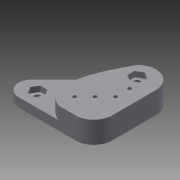
# Autodesk Inventor part: joint1+ax12imprint
Saved by Autodesk Inventor 2014 (Build 180170000, 170)
## iProperties
Created: 2014-01-13
Part Number: joint1+ax12imprint
Material: Générique
Document SubType Name: Modeling
Designer: helly
Density: 1 g/cm^3
Appearance: Par défaut
Author: helly
Autodesk Inventor part; units mm, degrees
ref_plane "YZ Plane" through (0, 0, 0) normal (1, 0, 0) x (0, 1, 0)
ref_plane "XZ Plane" through (0, 0, 0) normal (0, 1, 0) x (-1, 0, 0)
ref_plane "XY Plane" through (0, 0, 0) normal (0, 0, 1) x (1, 0, 0)
sketch "Esquisse1" plane through (0, 0, 0) normal (0, 0, 1) x (1, 0, 0)
  line L0 (0, 0) -> (52, 0) construction
  line L1 (0, 0) -> (25.4558, 25.4558) construction
  line L2 (0, 0) -> (-9.5459, 9.5459) construction
  line L3 (-9.5459, 9.5459) -> (-4.9497, 14.1421) construction
  line L4 (-4.9497, 14.1421) -> (0.7071, 19.799) construction
  line L5 (0.7071, 19.799) -> (6.364, 25.4558) construction
  line L6 (6.364, 25.4558) -> (12.0208, 31.1127) construction
  line L7 (25.4558, 25.4558) -> (19.799, 31.1127) construction
  line L8 (0, 0) -> (27.5772, 27.5772) construction
  circle A0 centre (0.7071, 19.799) radius 1 construction
  circle A1 centre (6.364, 25.4558) radius 1 construction
  circle A2 centre (12.0208, 31.1127) radius 1 construction
  circle A3 centre (19.799, 31.1127) radius 1 construction
  circle A4 centre (19.799, 0.7071) radius 1
  circle A5 centre (25.4558, 6.364) radius 1
  circle A6 centre (31.1127, 12.0208) radius 1
  circle A7 centre (31.1127, 19.799) radius 1
  circle A8 centre (27.5772, 27.5772) radius 2
  circle A9 centre (0, 0) radius 2
  line L9 (0, 0) -> (0, -8) construction
  line L10 (31.1127, 12.0208) -> (39.1127, 12.0208) construction
  line L11 (39.1127, 50.4264) -> (39.1127, -8)
  line L12 (0, 0) -> (-5.6569, 5.6569) construction
  line L13 (39.1127, -8) -> (-19.3137, -8)
  line L14 (-19.3137, -8) -> (39.1127, 50.4264)
  dimension "d31" = 45
  dimension "d32" = 13.5
  dimension "d33" = 6.5
  dimension "d34" = 8
  dimension "d35" = 8
  dimension "d36" = 8
  dimension "d37" = 8
  dimension "d38" = 36
  dimension "d39" = 39
  dimension "d40" = 2
  dimension "d41" = 4
  dimension "d44" = 8
  dimension "d45" = 8
  dimension "d64" = 8
  constraints: 30 end point, 10 centre point, 6 coincident, 6 perpendicular, 5 point on line, 4 collinear, 4 equal radius, 4 symmetric about line, 1 horizontal, 1 parallel, 4 other
  measures "d31" angle of L0 L1
  measures "d32" distance of L0.start L2.end
  measures "d33" distance of L2.end L3.end
  measures "d34" distance of L3.end L4.end
  measures "d35" distance of L4.end L5.end
  measures "d36" distance of L5.end L6.end
  measures "d37" distance of L1.end L7.end
  measures "d38" distance of L0.start L1.end
  measures "d39" distance of L0.start L8.end
  measures "d40" diameter of A0
  measures "d41" diameter of A8
  measures "d44" distance of L9.start L9.end
  measures "d45" distance of L10.start L10.end
  measures "d64" distance of L9.start L12.end
extrude "Extrusion7" add sketch "Esquisse1" along normal blind 12
sketch "Esquisse7" plane through (0, 0, 12) normal (0, 0, 1) x (1, 0, 0)
  circle A0 centre (0, 0) radius 2 projected
  circle A1 centre (27.5772, 27.5772) radius 2 projected
  circle A2 centre (19.799, 0.7071) radius 1 projected
  line L0 (39.1127, 50.4264) -> (-19.3137, -8) projected
  line L1 (-19.3137, -8) -> (39.1127, -8) projected
  circle A3 centre (0, 0) radius 12 construction
  circle A4 centre (19.799, 0.7071) radius 7.8116 construction
  circle A5 centre (27.5772, 27.5772) radius 8 construction
  line L2 (19.799, 0.7071) -> (19.799, -8) construction
  spline S0 degree 2 poles (19.799, -8) (2.3764, -1.7891) (21.9203, 33.234) knots 0 0 0 1 1 1
  point P0 (11.9924, 0.4283)
  dimension "d67" = 24
  constraints: 3 coincident, 2 end point, 2 point on line, 1 perpendicular, 13 other
extrude "Extrusion8" cut sketch "Esquisse7" against normal blind 7 contours S0 L1 L0
sketch "Esquisse8" plane through (0, 0, 5) normal (0, 0, 1) x (1, 0, 0)
  circle A0 centre (0, 0) radius 2 projected
  line L0 (19.799, -8) -> (-19.3137, -8) projected
  line L1 (4.0415, 0) -> (2.0207, -3.5)
  line L2 (2.0207, -3.5) -> (-2.0207, -3.5)
  line L3 (-2.0207, -3.5) -> (-4.0415, 0)
  line L4 (-4.0415, 0) -> (-2.0207, 3.5)
  line L5 (-2.0207, 3.5) -> (2.0207, 3.5)
  line L6 (2.0207, 3.5) -> (4.0415, 0)
  line L7 (2.0207, 3.5) -> (2.0207, -3.5) construction
  dimension "d70" = 7
  constraints: 14 end point, 1 coincident, 1 parallel, 1 perpendicular, 13 other
  measures "d70" distance of L5.end L1.end
extrude "Extrusion9" cut sketch "Esquisse8" against normal blind 3
sketch "Esquisse9" plane through (0, 0, 12) normal (0, 0, 1) x (1, 0, 0)
  line L0 (39.1127, -8) -> (39.1127, 50.4264) projected
  circle A0 centre (27.5772, 27.5772) radius 2 projected
  line L1 (31.0772, 29.5979) -> (31.0772, 25.5564)
  line L2 (31.0772, 25.5564) -> (27.5772, 23.5357)
  line L3 (27.5772, 23.5357) -> (24.0772, 25.5564)
  line L4 (24.0772, 25.5564) -> (24.0772, 29.5979)
  line L5 (24.0772, 29.5979) -> (27.5772, 31.6186)
  line L6 (27.5772, 31.6186) -> (31.0772, 29.5979)
  line L7 (24.0772, 29.5979) -> (31.0772, 29.5979) construction
  point P0 (0, 0)
  dimension "d73" = 7
  constraints: 14 end point, 1 coincident, 1 parallel, 13 other
  measures "d73" distance of L4.end L1.start
extrude "Extrusion10" cut sketch "Esquisse9" against normal blind 3
fillet "Congé2" radius 7 1 edges at (-19.3137, -8, 2.5)
fillet "Congé3" radius 10 1 edges at (39.1127, 50.4264, 6)
fillet "Congé4" radius 10 1 edges at (39.1127, -8, 6)
